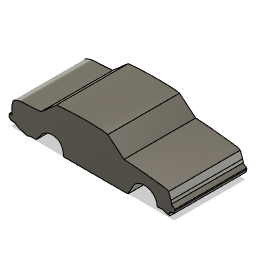
240 #MJP2022 v2 (Autodesk Fusion 360 design; units mm, degrees)
Autodesk Fusion 360 part; units mm, degrees
sketch "Sketch1" plane through (0, 0, 0) normal (0, 0, 1) x (1, 0, 0) in component "Chassi"
  line L0 (12.8004, -2.2692) -> (80.168, -2.2692)
  line L1 (0, 0) -> (12.8004, -2.2692)
  line L2 (0, 0) -> (80.168, 0)
  line L3 (80.168, -2.2692) -> (110.8391, 1.3227)
  spline S0 degree 5 poles (80.168, -2.2692) (80.2985, -2.0305) (80.558, -1.5551) (80.9427, -0.8476) (81.4465, 0.0842) (82.0614, 1.2294) (82.6617, 2.3538) (83.2486, 3.4549) (83.8238, 4.5284) (84.3901, 5.5682) (84.9511, 6.5656) (85.512, 7.509) (86.0783, 8.3863) (86.6549, 9.1865) (87.2452, 9.9021) (87.8506, 10.5309) (88.4688, 11.0785) (89.0943, 11.5583) (89.7228, 11.9866) (90.3533, 12.3786) (90.992, 12.7445) (91.6554, 13.0851) (92.3641, 13.3943) (93.1355, 13.6635) (93.9776, 13.8841) (94.8799, 14.0514) (95.8152, 14.166) (96.749, 14.2308) (97.6493, 14.2497) (98.4938, 14.226) (99.2812, 14.1603) (100.0317, 14.05) (100.7727, 13.8917) (101.529, 13.6822) (102.311, 13.4205) (103.1037, 13.1092) (103.8778, 12.7535) (104.601, 12.3603) (105.2481, 11.9365) (105.814, 11.4891) (106.3171, 11.0228) (106.7858, 10.5399) (107.2489, 10.0382) (107.7231, 9.5102) (108.2072, 8.9423) (108.6896, 8.3184) (109.1528, 7.6217) (109.5794, 6.8375) (109.9567, 5.9552) (110.2766, 4.9682) (110.5342, 3.8727) (110.6888, 2.9081) (110.7753, 2.1348) (110.82, 1.5971) (110.8391, 1.3227) knots 0 0 0 0 0 0 0.02 0.04 0.06 0.08 0.1 0.12 0.14 0.16 0.18 0.2 0.22 0.24 0.26 0.28 0.3 0.32 0.34 0.36 0.38 0.4 0.42 0.44 0.46 0.48 0.5 0.52 0.54 0.56 0.58 0.6 0.62 0.64 0.66 0.68 0.7 0.72 0.74 0.76 0.78 0.8 0.82 0.84 0.86 0.88 0.9 0.92 0.94 0.96 0.98 1 1 1 1 1 1
  line L4 (110.8391, 1.3227) -> (115.6138, 1.8819)
  line L5 (115.6138, 1.8819) -> (123.7732, -0.4732)
  line L6 (123.7732, -0.4732) -> (122.9623, 1.3227)
  line L7 (122.9623, 1.3227) -> (124.6855, 3.7009)
  line L8 (124.6855, 3.7009) -> (128.5611, 4.2197)
  line L9 (128.5611, 4.2197) -> (129.4571, 7.1067)
  line L10 (129.4571, 7.1067) -> (129.4571, 8.4332)
  line L11 (129.4571, 8.4332) -> (125.4178, 11.0302)
  line L12 (125.4178, 11.0302) -> (126.0292, 11.5506)
  line L13 (126.0292, 11.5506) -> (125.2284, 14.54)
  line L14 (125.2284, 14.54) -> (123.6315, 18.6804)
  line L15 (123.6315, 18.6804) -> (122.6811, 21.1444)
  spline S1 degree 5 poles (122.6811, 21.1444) (122.4084, 21.3011) (121.8261, 21.6003) (120.8421, 22.0064) (119.3059, 22.461) (117.0321, 22.8948) (114.4567, 23.2202) (111.7481, 23.5162) (108.9814, 23.8279) (106.1505, 24.169) (103.2075, 24.5357) (100.0857, 24.9143) (96.7347, 25.2924) (93.1294, 25.6623) (89.2589, 26.0193) (85.1232, 26.3609) (81.606, 26.6212) (78.8532, 26.809) (76.9673, 26.931) (76.0116, 26.9912) knots 0 0 0 0 0 0 0.066667 0.133333 0.2 0.266667 0.333333 0.4 0.466667 0.533333 0.6 0.666667 0.733333 0.8 0.866667 0.933333 1 1 1 1 1 1
  line L16 (76.0116, 26.9912) -> (59.1017, 41.0003)
  line L17 (120.2247, 22.4704) -> (110.3584, 23.7393)
  spline S2 degree 5 poles (59.1017, 41.0003) (58.7775, 41.0772) (58.1019, 41.225) (57.0068, 41.4293) (55.3827, 41.6666) (53.0826, 41.9047) (50.5293, 42.0856) (47.7613, 42.2129) (44.851, 42.2939) (41.8922, 42.3389) (38.981, 42.3584) (36.1989, 42.3618) (33.596, 42.3559) (31.1693, 42.3423) (28.8609, 42.3173) (26.5831, 42.2745) (24.2368, 42.2062) (21.7313, 42.1052) (19.0054, 41.9669) (16.0226, 41.7889) (12.7642, 41.5702) (9.9319, 41.3625) (7.6808, 41.1885) (6.124, 41.0644) (5.3315, 41.0003) knots 0 0 0 0 0 0 0.05 0.1 0.15 0.2 0.25 0.3 0.35 0.4 0.45 0.5 0.55 0.6 0.65 0.7 0.75 0.8 0.85 0.9 0.95 1 1 1 1 1 1
  line L18 (5.3315, 41.0003) -> (-10.7386, 26.8578)
  spline S3 degree 5 poles (-10.7386, 26.8578) (-11.2202, 26.8108) (-12.1734, 26.7195) (-13.5733, 26.5905) (-15.3799, 26.4344) (-17.5376, 26.266) (-19.5933, 26.1236) (-21.5449, 26.0059) (-23.3898, 25.9108) (-25.1249, 25.8345) (-26.7463, 25.7716) (-28.25, 25.7147) (-29.6312, 25.654) (-30.885, 25.5768) (-32.0083, 25.4701) (-33.0027, 25.3235) (-33.8774, 25.1319) (-34.6511, 24.8982) (-35.3569, 24.6372) (-36.0361, 24.3715) (-36.7228, 24.1185) (-37.4326, 23.8815) (-38.1452, 23.6353) (-38.8146, 23.3351) (-39.3921, 22.9365) (-39.8443, 22.4108) (-40.175, 21.7644) (-40.4135, 21.027) (-40.5997, 20.238) (-40.7704, 19.4335) (-40.9471, 18.6343) (-41.1017, 18.0076) (-41.2267, 17.5462) (-41.314, 17.2424) (-41.3587, 17.0915) knots 0 0 0 0 0 0 0.033333 0.066667 0.1 0.133333 0.166667 0.2 0.233333 0.266667 0.3 0.333333 0.366667 0.4 0.433333 0.466667 0.5 0.533333 0.566667 0.6 0.633333 0.666667 0.7 0.733333 0.766667 0.8 0.833333 0.866667 0.9 0.933333 0.966667 1 1 1 1 1 1
  line L19 (-41.3587, 17.0915) -> (-41.3587, 9.8396)
  line L20 (-41.3587, 9.8396) -> (-41.3587, 8.575)
  line L21 (-41.3587, 8.575) -> (-44.0429, 8.575)
  line L22 (-44.0429, 8.575) -> (-44.0429, 5.2768)
  line L23 (-44.0429, 5.2768) -> (-42.7008, 3.4751)
  line L24 (-42.7008, 3.4751) -> (-38.3746, 3.0146)
  line L25 (-38.3746, 3.0146) -> (-33.4921, 0.1131)
  line L26 (-33.4921, 0.1131) -> (-25.1399, -2.244)
  line L27 (-25.1399, -2.244) -> (-21.8112, -1.0654)
  line L28 (-21.8112, -1.0654) -> (-18.2433, -1.0654)
  line L29 (-18.2433, -1.0654) -> (-15.8469, -1.0654)
  spline S4 degree 5 poles (-15.8469, -1.0654) (-15.6741, -0.8323) (-15.3312, -0.3704) (-14.8252, 0.3088) (-14.1671, 1.1872) (-13.3718, 2.2397) (-12.6034, 3.2458) (-11.8605, 4.2039) (-11.1409, 5.1118) (-10.441, 5.966) (-9.7559, 6.762) (-9.0789, 7.4938) (-8.4026, 8.1563) (-7.7196, 8.7458) (-7.0227, 9.2618) (-6.3064, 9.7083) (-5.5665, 10.095) (-4.8009, 10.4335) (-4.0088, 10.7347) (-3.1909, 11.0056) (-2.3494, 11.2458) (-1.4875, 11.4478) (-0.6094, 11.6009) (0.2801, 11.6943) (1.1756, 11.7203) (2.0718, 11.678) (2.9629, 11.5717) (3.8425, 11.4082) (4.7034, 11.1942) (5.5373, 10.9336) (6.3345, 10.625) (7.0852, 10.2638) (7.7812, 9.8454) (8.417, 9.3669) (8.9914, 8.8309) (9.5081, 8.2451) (9.9732, 7.6191) (10.3938, 6.9611) (10.776, 6.2748) (11.1239, 5.5569) (11.4398, 4.8) (11.7249, 3.9941) (11.9797, 3.1295) (12.2044, 2.1988) (12.3993, 1.1974) (12.5648, 0.1227) (12.6737, -0.7967) (12.7422, -1.5198) (12.782, -2.0169) (12.8004, -2.2692) knots 0 0 0 0 0 0 0.022222 0.044444 0.066667 0.088889 0.111111 0.133333 0.155556 0.177778 0.2 0.222222 0.244444 0.266667 0.288889 0.311111 0.333333 0.355556 0.377778 0.4 0.422222 0.444444 0.466667 0.488889 0.511111 0.533333 0.555556 0.577778 0.6 0.622222 0.644444 0.666667 0.688889 0.711111 0.733333 0.755556 0.777778 0.8 0.822222 0.844444 0.866667 0.888889 0.911111 0.933333 0.955556 0.977778 1 1 1 1 1 1
  point P0 (84.3652, 5.515)
  point P1 (87.6184, 10.277)
  point P2 (90.4002, 12.3987)
  point P3 (93.5591, 13.766)
  point P4 (98.1103, 14.2312)
  point P5 (101.5272, 13.6717)
  point P6 (105.0001, 12.0885)
  point P7 (107.092, 10.2058)
  point P8 (109.1491, 7.5909)
  point P9 (115.2916, 23.1048)
  point P10 (101.6899, 24.7174)
  point P11 (49.8661, 42.106)
  point P12 (34.7789, 42.3575)
  point P13 (23.9663, 42.1899)
  point P14 (-28.3345, 25.709)
  point P15 (-34.2101, 25.0235)
  point P16 (-36.952, 24.0442)
  point P17 (-39.4002, 22.8691)
  point P18 (-40.5753, 20.323)
  point P19 (-10.6489, 5.7067)
  point P20 (-7.1109, 9.1803)
  point P21 (-3.6373, 10.8528)
  point P22 (0.4796, 11.6891)
  point P23 (4.7251, 11.1745)
  point P24 (8.1344, 9.5663)
  point P25 (10.3215, 7.0576)
  point P26 (11.8011, 3.7126)
  dimension "d1" = 13
  dimension "d2" = 10.052
  dimension "d5" = 67.3676
  dimension "d7" = 30.8807
  dimension "d8" = 173.321
  constraint horizontal L0
  constraint coincident L1.start L2.start
  constraint parallel L0 L2
  constraint parallel L3 L4
  constraint vertical L10
  constraint midpoint P9 L17
  constraint vertical L19
  constraint parallel L19 L20
  constraint perpendicular L20 L21
  constraint perpendicular L21 L22
  constraint horizontal L28
  constraint parallel L28 L29
  measures "d1" distance of L0.start L1.start
  measures "d2" angle of L1 L2
  measures "d5" distance of L0.start L0.end
  measures "d7" distance of L0.end L3.end
  measures "d8" angle of L0 L3
extrude "Extrude1" add sketch "Sketch1" along normal blind 75 contours L0 S0 L4 L5 L6 L7 L8 L9 L10 L11 L12 L13 L14 L15 S1 L16 S2 L18 S3 L19 L20 L21 L22 L23 L24 L25 L26 L27 L28 L29 S4 in component "Chassi"
component "Chassi" placed x (1, 0, 0) y (0, 1, 0) z (0, 0, 1) at (0, 0, 0)
